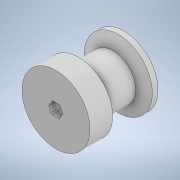
# Autodesk Inventor part: pulleyOneHalf
Saved by Autodesk Inventor 2020.2 (Build 242310000, 310)
## iProperties
Created: 2020-02-15
Part Number: pulleyOneHalf
Material: Generic
Document SubType Name: Modeling
Designer: robst
Density: 1 g/cm^3
Appearance: Default
Author: robst
Autodesk Inventor part; units mm, degrees
ref_plane "YZ Plane" through (0, 0, 0) normal (1, 0, 0) x (0, 1, 0)
ref_plane "XZ Plane" through (0, 0, 0) normal (0, 1, 0) x (-1, 0, 0)
ref_plane "XY Plane" through (0, 0, 0) normal (0, 0, 1) x (1, 0, 0)
sketch "Sketch1" plane through (0, 0, 0) normal (0, 0, 1) x (1, 0, 0)
  circle A0 centre (0, 0) radius 25.4
  line L0 (7.9189, 0) -> (3.9595, -6.858)
  line L1 (3.9595, -6.858) -> (-3.9595, -6.858)
  line L2 (-3.9595, -6.858) -> (-7.9189, 0)
  line L3 (-7.9189, 0) -> (-3.9595, 6.858)
  line L4 (-3.9595, 6.858) -> (3.9595, 6.858)
  line L5 (3.9595, 6.858) -> (7.9189, 0)
  dimension "d0" = 50.8
  dimension "d1" = 13.716
  constraints: 12 end point, 2 coincident, 1 centre point, 1 horizontal, 13 other
  measures "d0" diameter of A0
  measures "d1" distance between parallel lines of L1 L4
extrude "Extrusion1" add sketch "Sketch1" along normal mid plane 76.2
sketch "Sketch3" plane through (0, 0, 0) normal (1, 0, 0) x (0, 1, 0)
  line L0 (25.4, 38.1) -> (-25.4, 38.1) projected
  line L1 (25.4, 38.1) -> (38.1, 38.1)
  line L2 (25.4, -38.1) -> (25.4, 38.1) projected
  line L3 (0, -53.34) -> (0, 53.34) projected
  line L4 (38.1, 38.1) -> (38.1, 12.7)
  line L5 (38.1, 12.7) -> (24.2886, 6.2597)
  line L6 (24.2886, 6.2597) -> (25.4, 6.7779)
  line L7 (25.4, -38.1) -> (25.4, 38.1) projected
  point P0 (0, 0)
  point P1 (25.4, 19.4779)
  point P2 (25.4, 6.7779)
  dimension "d9" = 12.7
  dimension "d12" = 25.4
  dimension "d13" = 115
  constraints: 8 end point, 2 point on line, 1 collinear, 1 horizontal, 1 vertical
  measures "d9" distance of L0.start L1.end
  measures "d12" distance of L1.end L4.end
  measures "d13" angle of L4 L5
revolve "Revolution1" add sketch "Sketch3" angle 360 about axis through (0, 0, -10) along (0, 0, 1)
sketch "Sketch4" plane through (0, 0, 0) normal (1, 0, 0) x (0, 1, 0)
  line L0 (25.4, -38.1) -> (25.4, 6.7779) projected
  line L1 (-25.4, -38.1) -> (25.4, -38.1) projected
  line L2 (25.4, -38.1) -> (38.1, -38.1)
  line L3 (38.1, -38.1) -> (38.1, -31.75)
  line L4 (38.1, -31.75) -> (24.8707, -25.5811)
  line L5 (0, -46.9275) -> (0, 14.8652) projected
  line L6 (24.8707, -25.5811) -> (25.4, -25.8279)
  line L7 (25.4, -38.1) -> (25.4, 6.7779) projected
  point P0 (0, 0)
  point P1 (25.4, -25.8279)
  dimension "d14" = 12.7
  dimension "d15" = 6.35
  dimension "d16" = 115
  constraints: 8 end point, 1 collinear, 1 horizontal, 1 perpendicular, 1 point on line
  measures "d14" distance of L0.start L2.end
  measures "d15" distance of L2.end L3.end
  measures "d16" angle of L4 L3
revolve "Revolution2" add sketch "Sketch4" angle 360 about axis through (0, 0, -10) along (0, 0, 1)
body "Solid1"
